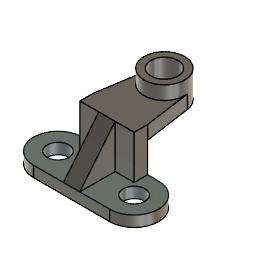
EX-2.2 (Autodesk Fusion 360 design; units mm, degrees)
part number: 2026-05-02-13-26-49-903
Autodesk Fusion 360 part; units mm, degrees
sketch "Sketch1" plane through (0, 0, 0) normal (0, 0, 1) x (1, 0, 0)
  circle A0 centre (-28, 0) radius 8
  line L0 (0, 0) -> (0, 62.0025)
  circle A1 centre (28, 0) radius 8
  line L1 (-28, 18) -> (28, 18)
  line L2 (-28, -18) -> (28, -18)
  arc A2 (28, -18) -> (28, 18) centre (28, 0) ccw
  arc A3 (-28, 18) -> (-28, -18) centre (-28, 0) ccw
  dimension "d1" = 16
  dimension "d2" = 36
  dimension "d3" = 28
  constraint concentric A0 A3
  constraint coincident L0.start origin
  constraint vertical L0
  constraint symmetric A0 L0 A1
  constraint symmetric L0 A2 A3
  constraint horizontal L1
  constraint horizontal L2
  constraint tangent L1 A3
  constraint tangent L2 A3
  measures "d1" diameter of A0
  measures "d2" diameter of A3
  measures "d3" distance of L0.start A0.centre
extrude "Extrude1" add sketch "Sketch1" along normal blind 8
sketch "Sketch2" plane through (0, 0, 8) normal (0, 0, 1) x (-1, 0, 0)
  circle A0 centre (28, 0) radius 8
  circle A1 centre (-28, 0) radius 8
  arc A2 (28, -18) -> (28, 18) centre (28, 0) ccw
  line L0 (28, 18) -> (-28, 18)
  arc A3 (-28, 18) -> (-28, -18) centre (-28, 0) ccw
  line L1 (-28, -18) -> (28, -18)
sketch "Sketch3" plane through (0, 0, 8) normal (0, 0, 1) x (-1, 0, 0)
  line L0 (20, -18) -> (-20, -18)
  line L1 (-20, -18) -> (-20, -8)
  line L2 (-20, -8) -> (20, -8)
  line L3 (20, -8) -> (20, -18)
  dimension "d6" = 40
  dimension "d7" = 10
  dimension "d8" = 20
  constraint horizontal L0
  constraint vertical L1
  constraint horizontal L2
  constraint vertical L3
  measures "d6" distance of L0.start L0.end
  measures "d7" distance of L0.start L2.end
  measures "d8" distance of L3 origin
extrude "Extrude2" add sketch "Sketch3" along normal blind 32
sketch "Sketch4" plane through (0, 0, 40) normal (0, 0, 1) x (-1, 0, 0)
  line L0 (20, -8) -> (-20, -8)
  line L1 (-20, -8) -> (-20, -18)
  line L2 (-20, -18) -> (20, -18)
  line L3 (20, -18) -> (20, -8)
  circle A0 centre (-0.2889, -50) radius 10
  line L4 (14.5242, -52.3607) -> (20, -18)
  line L5 (-15.1389, -52.1159) -> (-20, -18)
  arc A1 (-15.1389, -52.1159) -> (14.5242, -52.3607) centre (-0.2889, -50) ccw
  dimension "d11" = 20
  dimension "d12" = 30
  dimension "d13" = 32
  constraint concentric A0 A1
  constraint tangent L4 A1
  constraint coincident L2.end L3.start
  constraint tangent L5 A1
  constraint coincident L1.end L2.start
  measures "d11" diameter of A0
  measures "d12" diameter of A1
  measures "d13" distance of L2 A0.centre
extrude "Extrude3" add sketch "Sketch4" against normal blind 10 contours L2 L4 L5 A1
sketch "Sketch5" plane through (0, 0, 40) normal (0, 0, 1) x (-1, 0, 0)
  circle A0 centre (-0.2889, -50) radius 10
  line L0 (20, -8) -> (-20, -8)
  line L1 (-20, -8) -> (-20, -18)
  line L2 (-20, -18) -> (-15.1389, -52.1159)
  arc A1 (-15.1389, -52.1159) -> (14.5242, -52.3607) centre (-0.2889, -50) ccw
  line L3 (14.5242, -52.3607) -> (20, -18)
  line L4 (20, -18) -> (20, -8)
  circle A2 centre (-0.2889, -50) radius 10
  circle A3 centre (-0.2889, -50) radius 15
  dimension "d16" = 20
  dimension "d17" = 30
  constraint concentric A0 A2
  constraint concentric A2 A3
  measures "d16" diameter of A2
  measures "d17" diameter of A3
extrude "Extrude4" add sketch "Sketch5" along normal blind 10 contours A1 A3
sketch "Sketch6" plane through (0, 0, 0) normal (1, 0, 0) x (0, 1, 0)
  line L0 (8, 40, -20) -> (8, 40, 20)
  line L1 (-18, 8, -28) -> (-18, 8, 28)
  line L2 (8, 40) -> (-18, 8)
  line L3 (8, 8, 20) -> (8, 8, -20)
  line L4 (-18, 8) -> (8, 8)
  line L5 (8, 40) -> (8, 8)
extrude "Extrude5" add sketch "Sketch6" along normal blind 6 and the other way blind 6
